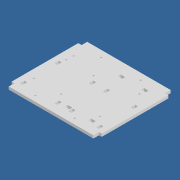
# Autodesk Inventor part: BoardCarrier
Saved by Autodesk Inventor 2021 (Build 250183000, 183)
## iProperties
Created: 2022-09-21
Part Number: BoardCarrier
Material: Generic
Document SubType Name: Modeling
Designer: Nathann
Density: 1 g/cm^3
Appearance: Default
Author: Nathann
Autodesk Inventor part; units mm, degrees
ref_plane "YZ Plane" through (0, 0, 0) normal (1, 0, 0) x (0, 1, 0)
ref_plane "XZ Plane" through (0, 0, 0) normal (0, 1, 0) x (-1, 0, 0)
ref_plane "XY Plane" through (0, 0, 0) normal (0, 0, 1) x (1, 0, 0)
sketch "Sketch1" plane through (0, 0, 0) normal (0, 1, 0) x (-1, 0, 0)
  line L0 (0, 0) -> (162, 0)
  line L1 (162, 0) -> (162, 120)
  line L2 (162, 120) -> (0, 120)
  line L3 (0, 120) -> (0, 0)
  line L4 (157, 120) -> (5, 120)
  line L5 (5, 120) -> (5, 130)
  line L6 (5, 130) -> (157, 130)
  line L7 (157, 130) -> (157, 120)
  line L8 (156, 0) -> (6, 0)
  line L9 (6, 0) -> (6, -10)
  line L10 (6, -10) -> (156, -10)
  line L11 (156, -10) -> (156, 0)
  dimension "d0" = 120
  dimension "d1" = 162
  dimension "d2" = 5
  dimension "d3" = 5
  dimension "d4" = 10
  dimension "d5" = 10
  dimension "d6" = 150
  constraints: 24 end point, 6 parallel, 3 horizontal, 3 perpendicular, 2 point on line
  measures "d0" distance of L2.end L0.start
  measures "d1" distance of L0.start L0.end
  measures "d2" distance between parallel lines of L1 L7
  measures "d3" distance between parallel lines of L3 L5
  measures "d4" distance of L6.end L4.start
  measures "d5" distance of L10.end L8.start
  measures "d6" distance of L9.end L10.end
extrude "Extrusion1" add sketch "Sketch1" along normal blind 5
sketch "Sketch2" plane through (0, 5, 0) normal (0, 1, 0) x (1, 0, 0)
  circle A0 centre (-147, -37) radius 1.5444
  circle A1 centre (-98, -37) radius 1.5
  circle A2 centre (-98, -95) radius 1.5
  circle A3 centre (-147, -95) radius 1.5
  circle A4 centre (-28.0426, -24.3) radius 1.5
  circle A5 centre (-146.3426, -24.3) radius 1.5
  circle A6 centre (-28.7, -95) radius 1.5
  line L0 (-75, -105.8843) -> (-67, -105.8843)
  line L1 (-67, -105.8843) -> (-67, -110.8843)
  line L2 (-67, -110.8843) -> (-75, -110.8843)
  line L3 (-75, -110.8843) -> (-75, -105.8843)
  line L4 (-75, -10.8843) -> (-67, -10.8843)
  line L5 (-67, -10.8843) -> (-67, -15.8843)
  line L6 (-67, -15.8843) -> (-75, -15.8843)
  line L7 (-75, -15.8843) -> (-75, -10.8843)
  line L8 (-25, -10.8843) -> (-33, -10.8843)
  line L9 (-33, -10.8843) -> (-33, -15.8843)
  line L10 (-33, -15.8843) -> (-25, -15.8843)
  line L11 (-25, -15.8843) -> (-25, -10.8843)
  line L12 (-25, -105.8843) -> (-33, -105.8843)
  line L13 (-33, -105.8843) -> (-33, -110.8843)
  line L14 (-33, -110.8843) -> (-25, -110.8843)
  line L15 (-25, -110.8843) -> (-25, -105.8843)
  line L16 (-15, -45) -> (-10, -45)
  line L17 (-10, -45) -> (-10, -53)
  line L18 (-10, -53) -> (-15, -53)
  line L19 (-15, -53) -> (-15, -45)
  line L20 (-65, -45) -> (-60, -45)
  line L21 (-60, -45) -> (-60, -53)
  line L22 (-60, -53) -> (-65, -53)
  line L23 (-65, -53) -> (-65, -45)
  line L24 (-60, -107) -> (-65, -107)
  line L25 (-65, -107) -> (-65, -115)
  line L26 (-65, -115) -> (-60, -115)
  line L27 (-60, -115) -> (-60, -107)
  line L28 (-10, -107) -> (-15, -107)
  line L29 (-15, -107) -> (-15, -115)
  line L30 (-15, -115) -> (-10, -115)
  line L31 (-10, -115) -> (-10, -107)
  line L32 (-162, 0) -> (-162, -120) projected
  line L33 (-157, -130) -> (-5, -130) projected
  line L34 (0, -120) -> (0, 0) projected
  line L35 (-152, -107) -> (-147, -107)
  line L36 (-147, -107) -> (-147, -115)
  line L37 (-147, -115) -> (-152, -115)
  line L38 (-152, -115) -> (-152, -107)
  line L39 (-147, -45) -> (-152, -45)
  line L40 (-152, -45) -> (-152, -53)
  line L41 (-152, -53) -> (-147, -53)
  line L42 (-147, -53) -> (-147, -45)
  line L43 (-90.0773, -45) -> (-85.0773, -45)
  line L44 (-85.0773, -45) -> (-85.0773, -53)
  line L45 (-85.0773, -53) -> (-90.0773, -53)
  line L46 (-90.0773, -53) -> (-90.0773, -45)
  line L47 (-85, -107) -> (-90, -107)
  line L48 (-90, -107) -> (-90, -115)
  line L49 (-90, -115) -> (-85, -115)
  line L50 (-85, -115) -> (-85, -107)
  dimension "d9" = 3
  dimension "d10" = 15
  dimension "d11" = 58
  dimension "d12" = 49
  dimension "d13" = 49
  dimension "d14" = 58
  dimension "d15" = 3
  dimension "d16" = 3
  dimension "d17" = 3.0888
  dimension "d18" = 35
  dimension "d19" = 70.7
  dimension "d20" = 118.3
  dimension "d21" = 70.7
  dimension "d22" = 118.3
  dimension "d23" = 3
  dimension "d24" = 3
  dimension "d25" = 3
  dimension "d26" = 5
  dimension "d27" = 8
  dimension "d28" = 8
  dimension "d29" = 5
  dimension "d30" = 8
  dimension "d31" = 5
  dimension "d32" = 5
  dimension "d33" = 8
  dimension "d34" = 8
  dimension "d35" = 5
  dimension "d36" = 5
  dimension "d37" = 8
  dimension "d38" = 8
  dimension "d39" = 5
  dimension "d40" = 5
  dimension "d41" = 8
  dimension "d42" = 50
  dimension "d43" = 25
  dimension "d44" = 50
  dimension "d45" = 25
  dimension "d46" = 90
  dimension "d47" = 90
  dimension "d48" = 55
  dimension "d49" = 55
  dimension "d50" = 70
  dimension "d51" = 70
  dimension "d52" = 10
  dimension "d55" = 35
  dimension "d56" = 15
  dimension "d57" = 15
  dimension "d58" = 8
  dimension "d59" = 10
  dimension "d60" = 5
  dimension "d61" = 5
  dimension "d62" = 8
  dimension "d63" = 10
  dimension "d64" = 70
  dimension "d65" = 5
  dimension "d66" = 5
  dimension "d67" = 8
  dimension "d68" = 8
  dimension "d69" = 70
  dimension "d70" = 0
  dimension "d71" = 0
  constraints: 96 end point, 24 parallel, 12 horizontal, 12 perpendicular, 7 centre point, 7 point on line, 1 horizontal alignment, 1 vertical alignment
  measures "d9" diameter of A3
  measures "d10" distance from line of L32 A3.centre
  measures "d11" distance of A3.centre A0.centre
  measures "d12" distance of A0.centre A1.centre
  measures "d13" distance of A3.centre A2.centre
  measures "d14" distance of A2.centre A1.centre
  measures "d15" diameter of A2
  measures "d16" diameter of A1
  measures "d17" diameter of A0
  measures "d18" distance from line of L33 A3.centre
  measures "d19" vertical distance of A3.centre A5.centre
  measures "d20" distance of A6.centre A3.centre
  measures "d21" vertical distance of A4.centre A6.centre
  measures "d22" distance of A5.centre A4.centre
  measures "d23" diameter of A4
  measures "d24" diameter of A6
  measures "d25" diameter of A5
  measures "d26" distance of L16.start L16.end
  measures "d27" distance of L16.end L17.end
  measures "d28" distance of L30.end L28.start
  measures "d29" distance of L29.end L30.end
  measures "d30" distance of L13.end L14.end
  measures "d31" distance of L14.end L12.start
  measures "d32" distance of L0.end L1.end
  measures "d33" distance of L1.end L2.end
  measures "d34" distance of L26.end L24.start
  measures "d35" distance of L25.end L26.end
  measures "d36" distance of L21.end L22.end
  measures "d37" distance of L22.end L20.start
  measures "d38" distance of L5.end L6.end
  measures "d39" distance of L6.end L4.start
  measures "d40" distance of L10.end L8.start
  measures "d41" distance of L8.start L8.end
  measures "d42" distance between parallel lines of L11 L7
  measures "d43" distance between parallel lines of L34 L11
  measures "d44" distance between parallel lines of L15 L3
  measures "d45" distance between parallel lines of L34 L15
  measures "d46" distance between parallel lines of L0 L6
  measures "d47" distance between parallel lines of L12 L10
  measures "d48" distance between parallel lines of L17 L23
  measures "d49" distance between parallel lines of L31 L25
  measures "d50" distance between parallel lines of L16 L30
  measures "d51" distance between parallel lines of L26 L20
  measures "d52" distance between parallel lines of L34 L17
  measures "d55" distance from line of L33 A6.centre
  measures "d56" distance between parallel lines of L33 L30
  measures "d57" distance between parallel lines of L37 L33
  measures "d58" distance of L37.end L35.start
  measures "d59" distance between parallel lines of L32 L38
  measures "d60" distance of L35.start L35.end
  measures "d61" distance of L40.end L41.end
  measures "d62" distance of L41.end L39.start
  measures "d63" distance between parallel lines of L32 L40
  measures "d64" distance between parallel lines of L39 L37
  measures "d65" distance of L47.start L47.end
  measures "d66" distance of L44.end L45.end
  measures "d67" distance of L43.end L44.end
  measures "d68" distance of L47.end L48.end
  measures "d69" distance between parallel lines of L50 L29
  measures "d70" distance between parallel lines of L49 L30
  measures "d71" distance between parallel lines of L45 L18
extrude "Extrusion2" cut sketch "Sketch2" against normal mid plane 40
sketch "Sketch4" plane through (0, 5, 0) normal (0, 1, 0) x (1, 0, 0)
  circle A0 centre (-48.4143, -2) radius 1.5
  circle A1 centre (-119.1143, -2) radius 1.5
  circle A2 centre (-119.1143, -120.3) radius 1.5
  circle A3 centre (-48.4143, -120.3) radius 1.5
  circle A4 centre (-146.3426, -24.3) radius 1.5 projected
  circle A5 centre (-28.0426, -24.3) radius 1.5 projected
  circle A6 centre (-28.7, -95) radius 1.5 projected
  line L0 (-6, 10) -> (-156, 10) projected
  point P0 (0, 0)
  dimension "d72" = 118.3
  dimension "d73" = 70.7
  dimension "d74" = 118.3
  dimension "d75" = 70.7
  dimension "d76" = 70.7
  dimension "d77" = 118.3
  dimension "d78" = 3
  dimension "d79" = 3
  dimension "d80" = 3
  dimension "d81" = 3
  dimension "d82" = 3
  dimension "d83" = 12
  dimension "d84" = 12
  constraints: 4 centre point, 1 vertical alignment
  measures "d72" distance of A4.centre A5.centre
  measures "d73" vertical distance of A5.centre A6.centre
  measures "d74" distance of A3.centre A0.centre
  measures "d75" distance of A1.centre A0.centre
  measures "d76" distance of A2.centre A3.centre
  measures "d77" distance of A1.centre A2.centre
  measures "d78" diameter of A0
  measures "d79" diameter of A5
  measures "d80" diameter of A3
  measures "d81" diameter of A2
  measures "d82" diameter of A1
  measures "d83" distance from line of L0 A0.centre
  measures "d84" distance from line of L0 A1.centre
extrude "Extrusion3" cut sketch "Sketch4" against normal mid plane 30 contours A0 | A1 | A2 | A3
equation "\"d2\" = d3"
equation "\"d3\" = WoodWidth"
equation "\"d7\" = WoodWidth"
equation "\"d14\" = d11"
equation "\"d16\" = d15"
equation "\"d21\" = d19"
equation "\"d22\" = d20"
equation "\"d23\" = d9"
equation "\"d24\" = d9"
equation "\"d25\" = d9"
equation "\"d45\" = d43"
equation "\"d55\" = d18"
equation "\"d57\" = d56"
equation "\"d74\" = d72"
equation "\"d75\" = d73"
equation "\"d76\" = d75"
equation "\"d77\" = d74"
equation "\"d78\" = d79"
equation "\"d80\" = d78"
equation "\"d81\" = d78"
equation "\"d82\" = d78"
equation "\"d84\" = d83"
equation "\"WoodWidth\" = 5"
equation "\"LaserWith\" = 0.3"
body "Solid1"
